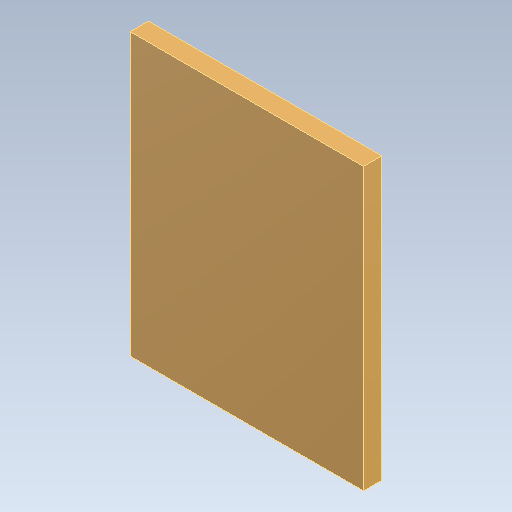
# Autodesk Inventor part: BGM220P
Saved by Autodesk Inventor 2021 (Build 250183000, 183)
## iProperties
Created: 2020-11-03
Part Number: BGM220P
Material: Generic
Document SubType Name: Modeling
Designer: faiya
Density: 1 g/cm^3
Appearance: BGM220P, BGM220P
Author: faiya
Autodesk Inventor part; units mm, degrees
ref_plane "YZ Plane" through (0, 0, 0) normal (1, 0, 0) x (0, 1, 0)
ref_plane "XZ Plane" through (0, 0, 0) normal (0, 1, 0) x (-1, 0, 0)
ref_plane "XY Plane" through (0, 0, 0) normal (0, 0, 1) x (1, 0, 0)
sketch "BGM220P, BGM220P_6" plane through (0, 0, 0) normal (0, 0, 1) x (1, 0, 0)
  line L0 (-0.0635, 6.4135) -> (12.7, 6.4135)
  line L1 (12.7, 6.4135) -> (12.7, -8.9535)
  line L2 (12.7, -8.9535) -> (-0.0635, -8.9535)
  line L3 (-0.0635, -8.9535) -> (-0.0635, 6.4135)
  constraints: 8 end point
extrude "Extrusion1" add sketch "BGM220P, BGM220P_6" along normal blind 1
body "Solid1"
